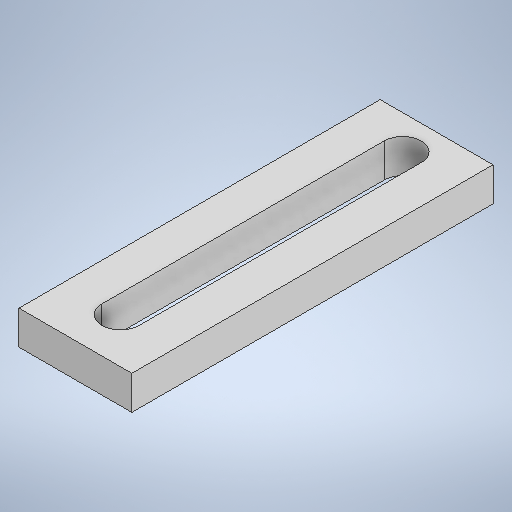
# Autodesk Inventor part: BeltMount2
Saved by Autodesk Inventor 2025.2 (Build 292293000, 293)
## iProperties
Created: 2025-07-29
Part Number: BeltMount2
Material: Generic
Document SubType Name: Modeling
Designer: Simon
Density: 1 g/cm^3
Appearance: Default
Author: Simon
Autodesk Inventor part; units mm, degrees
ref_plane "YZ Plane" through (0, 0, 0) normal (1, 0, 0) x (0, 1, 0)
ref_plane "XZ Plane" through (0, 0, 0) normal (0, 1, 0) x (-1, 0, 0)
ref_plane "XY Plane" through (0, 0, 0) normal (0, 0, 1) x (1, 0, 0)
sketch "Sketch1" plane through (0, 0, 0) normal (0, 1, 0) x (-1, 0, 0)
  line L0 (0, 0) -> (10, 0)
  line L1 (10, 0) -> (10, -32)
  line L2 (10, -32) -> (0, -32)
  line L3 (0, -32) -> (0, 0)
  line L4 (5, 0) -> (5, -4)
  line L5 (5, -32) -> (5, -29)
  line L6 (5, -4) -> (5, -29) construction
  line L7 (3.35, -4) -> (3.35, -29)
  line L8 (6.65, -29) -> (6.65, -4)
  arc A0 (6.65, -4) -> (3.35, -4) centre (5, -4) ccw
  arc A1 (3.35, -29) -> (6.65, -29) centre (5, -29) ccw
  point P0 (5, -16.5)
  dimension "d0" = 10
  dimension "d1" = 32
  dimension "d2" = 4
  dimension "d3" = 3
  dimension "d4" = 3.3
  constraints: 20 end point, 4 point on circle, 4 tangent, 3 midpoint, 3 parallel, 2 centre point, 2 vertical, 1 collinear, 1 horizontal, 1 perpendicular
  measures "d0" distance of L1.end L2.end
  measures "d1" distance of L0.end L1.end
  measures "d2" distance of L4.start L4.end
  measures "d3" distance of L5.start L5.end
  measures "d4" diameter of A1
extrude "Extrusion1" add sketch "Sketch1" along normal blind 3 contours L0 L4 A0 L7 A1 L5 L2 L3 | L0 L1 L2 L5 A1 L8 A0 L4
body "Solid1"
